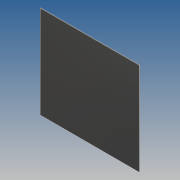
# Autodesk Inventor part: Front_Cover_V1
Saved by Autodesk Inventor 2019 (Build 230136000, 136)
## iProperties
Created: 2020-08-28
Part Number: Front_Cover_V1
Material: Generic
Document SubType Name: Modeling
Designer: voigt
Density: 1 g/cm^3
Appearance: Dark Gray
Author: voigt
Autodesk Inventor part; units mm, degrees
ref_plane "YZ Plane" through (0, 0, 0) normal (1, 0, 0) x (0, 1, 0)
ref_plane "XZ Plane" through (0, 0, 0) normal (0, 1, 0) x (-1, 0, 0)
ref_plane "XY Plane" through (0, 0, 0) normal (0, 0, 1) x (1, 0, 0)
sketch "Sketch1" plane through (0, 0, 0) normal (0, 0, 1) x (1, 0, 0)
  line L0 (0, 253.4) -> (0, -253.4) construction
  line L1 (-270.9, 0) -> (270.9, 0) construction
  line L2 (-193.5, 181) -> (193.5, 181)
  line L3 (193.5, 181) -> (193.5, -181)
  line L4 (193.5, -181) -> (-193.5, -181)
  line L5 (-193.5, -181) -> (-193.5, 181)
  point P0 (0, 0)
  dimension "d0" = 362
  dimension "d1" = 387
  constraints: 8 end point, 2 parallel, 1 horizontal, 1 perpendicular, 2 other
  measures "d0" distance of L4.end L2.start
  measures "d1" distance of L2.start L2.end
extrude "Extrusion1" add sketch "Sketch1" along normal blind 2
body "Solid1"
